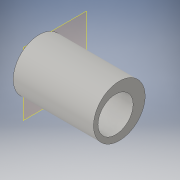
# Autodesk Inventor part: Part2
Saved by Autodesk Inventor 2016 (Build 200138000, 138)
## iProperties
Created: 2018-04-05
Part Number: Part2
Material: Generic
Document SubType Name: Modeling
Designer: User
Density: 1 g/cm^3
Appearance: Default
Project: Project_2
Cost Center: €2.00
Catalog Web Link: www.cork.ie
Description: Element2
Vendor: Cork
Engineer: MasterBlaster
Authority: TeamLeader
Stock Number: 8753
Author: User
Revision Number: s09760
Autodesk Inventor part; units mm, degrees
ref_plane "XZ Plane" through (0, 0, 0) normal (0, 1, 0) x (-1, 0, 0)
ref_plane "XY Plane" through (0, 0, 0) normal (0, 0, 1) x (1, 0, 0)
ref_plane "Work Plane1" through (11.1125, 0, 0) normal (1, 0, 0) x (0, 1, 0)
sketch "Sketch1" plane through (11.1125, 0, 0) normal (1, 0, 0) x (0, 1, 0)
  circle A0 centre (2.8405, 5.0014) radius 8.1634
  arc A1 (4.3899, 0) -> (1.128, -3.1259) centre (-0.2391, 1.5655) ccw
  point P0 (0, 0)
  constraints: 2 centre point, 2 point on circle
extrude "Extrusion1" add sketch "Sketch1" along normal blind 25.4
hole "Hole1" at (36.5125, 2.4608, 6.2031) direction (-1, 0, 0) diameter 11.1125 end through all
body "Solid1"
